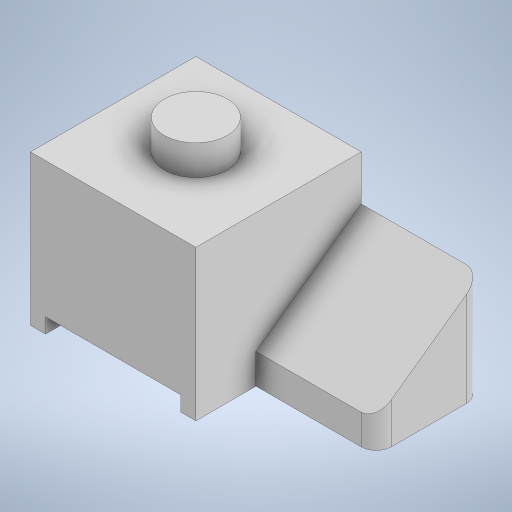
# Autodesk Inventor part: khurramf_Graphics2
Saved by Autodesk Inventor 2024 (Build 280153000, 153)
## iProperties
Created: 2023-09-15
Part Number: khurramf_Graphics2
Material: Generic
Document SubType Name: Modeling
Designer: furqa
Density: 1 g/cm^3
Appearance: Default
Author: furqa
Autodesk Inventor part; units mm, degrees
ref_plane "YZ Plane" through (0, 0, 0) normal (1, 0, 0) x (0, 1, 0)
ref_plane "XZ Plane" through (0, 0, 0) normal (0, 1, 0) x (-1, 0, 0)
ref_plane "XY Plane" through (0, 0, 0) normal (0, 0, 1) x (1, 0, 0)
sketch "Sketch1" plane through (0, 0, 0) normal (0, 0, 1) x (1, 0, 0)
  line L0 (0, 0) -> (5, 0)
  line L1 (5, 0) -> (5, 5)
  line L2 (5, 5) -> (50, 5)
  line L3 (50, 5) -> (50, 0)
  line L4 (50, 0) -> (55, 0)
  line L5 (55, 0) -> (55, 50)
  line L6 (55, 50) -> (0, 50)
  line L7 (0, 50) -> (0, 0)
  dimension "d0" = 50
  dimension "d1" = 5
  dimension "d2" = 5
  dimension "d3" = 5
  dimension "d4" = 45
  constraints: 16 end point, 6 perpendicular, 2 point on line, 1 horizontal
  measures "d0" distance of L6.end L0.start
  measures "d1" distance of L0.end L1.end
  measures "d2" distance of L0.start L0.end
  measures "d3" distance of L3.end L4.end
  measures "d4" distance of L1.end L2.end
extrude "Extrusion1" add sketch "Sketch1" along normal blind 55
sketch "Sketch2" plane through (0, 50, 0) normal (0, 1, 0) x (1, 0, 0)
  circle A0 centre (27.5, -27.5) radius 10.5
  line L0 (55, -55) -> (0, -55) projected
  line L1 (0, 0) -> (0, -55) projected
  dimension "d7" = 21
  dimension "d8" = 27.5
  dimension "d9" = 27.5
  constraints: 1 centre point
  measures "d7" diameter of A0
  measures "d8" distance from line of L0 A0.centre
  measures "d9" distance from line of L1 A0.centre
extrude "Extrusion2" add sketch "Sketch2" along normal blind 10
sketch "Sketch3" plane through (55, 0, 0) normal (1, 0, 0) x (0, 0, -1)
  line L0 (0, 50) -> (0, 0) projected
  line L1 (0, 0) -> (0, 35)
  line L2 (0, 35) -> (-35, 10)
  line L3 (-35, 10) -> (-35, 0)
  line L4 (0, 0) -> (-55, 0) projected
  line L5 (-35, 0) -> (0, 0)
  line L6 (0, 0) -> (0, 35)
  point P0 (-35, 0)
  dimension "d12" = 35
  dimension "d13" = 0
  dimension "d14" = 10
  dimension "d15" = 35
  constraints: 10 end point, 2 perpendicular, 2 point on line, 1 collinear
  measures "d12" distance of L5.end L1.end
  measures "d13" distance between parallel lines of L4 L5
  measures "d14" distance of L2.end L3.end
  measures "d15" distance of L0.end L3.end
extrude "Extrusion3" add sketch "Sketch3" along normal blind 40
fillet "Fillet1" radius 5 1 edges at (95, 5, 35)
fillet "Fillet2" radius 5 1 edges at (95, 17.5, 0)
body "Solid1"
